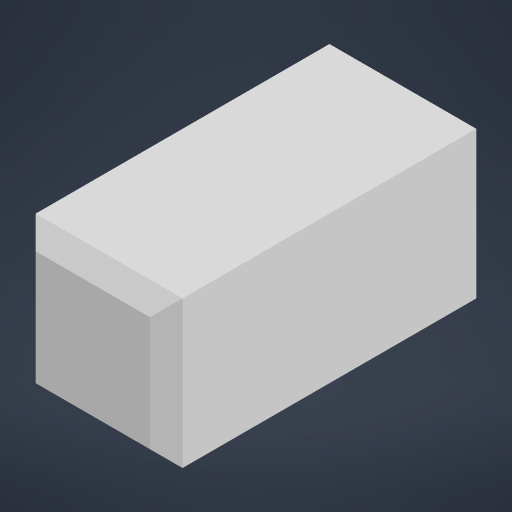
# Autodesk Inventor part: Pillar_TestFit_V1
Saved by Autodesk Inventor 2024 (Build 280153000, 153)
## iProperties
Created: 2023-07-01
Part Number: Pillar_TestFit_V1
Material: Generic
Document SubType Name: Modeling
Designer: User
Density: 1 g/cm^3
Appearance: Default
Author: User
Autodesk Inventor part; units mm, degrees
ref_plane "YZ Plane" through (0, 0, 0) normal (1, 0, 0) x (0, 1, 0)
ref_plane "XZ Plane" through (0, 0, 0) normal (0, 1, 0) x (-1, 0, 0)
ref_plane "XY Plane" through (0, 0, 0) normal (0, 0, 1) x (1, 0, 0)
sketch "Sketch1" plane through (0, 0, 0) normal (0, 0, 1) x (1, 0, 0)
  line L0 (0, 0) -> (-9, 0)
  line L1 (-9, 0) -> (-9, 9)
  line L2 (-9, 9) -> (0, 9)
  line L3 (0, 9) -> (0, 0)
  dimension "d0" = 9
  dimension "d1" = 9
  constraints: 8 end point, 2 parallel, 1 horizontal, 1 perpendicular
  measures "d0" distance of L1.end L2.end
  measures "d1" distance of L0.end L1.end
extrude "Extrusion1" add sketch "Sketch1" along normal blind 20
chamfer "Chamfer1" distance 1 angle 45 4 edges at (-4.5, 9, 20) (0, 4.5, 20) (-4.5, 0, 20) (-9, 4.5, 20)
chamfer "Chamfer2" distance 1 angle 45 4 edges at (-4.5, 9, 0) (0, 4.5, 0) (-4.5, 0, 0) (-9, 4.5, 0)
body "Solid1"
